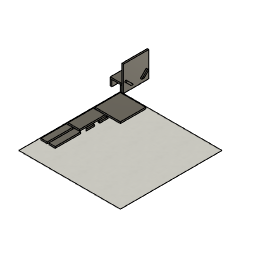
SplineJigV1 (Autodesk Fusion 360 design; units mm, degrees)
Autodesk Fusion 360 part; units mm, degrees
sketch "Sketch2" plane through (0, 0, 0) normal (1, 0, 0) x (0, 1, 0)
  line L0 (0, 0) -> (304.8, 0)
  line L1 (304.8, 0) -> (304.8, 76.2)
  line L2 (304.8, 76.2) -> (0, 76.2)
  line L3 (0, 76.2) -> (0, 0)
  dimension "d1" = 304.8
  dimension "d2" = 76.2
  constraint horizontal L0
  constraint vertical L1
  constraint horizontal L2
  constraint vertical L3
  constraint coincident L0.start L3.end
  measures "d1" distance of L0.start L0.end
  measures "d2" distance of L0.start L2.end
extrude "Extrude1" add sketch "Sketch2" along normal blind 18 makes body 1
sketch "Sketch5" plane through (0, 0, 76.2) normal (0, 0, 1) x (-1, 0, 0)
  line L0 (0, -304.8) -> (0, 0)
  line L1 (0, 0) -> (-18, 0)
  line L2 (-18, 0) -> (-18, -304.8)
  line L3 (-18, -304.8) -> (0, -304.8)
  line L4 (-18, -304.8) -> (121.1875, -304.8)
  line L5 (121.1875, -304.8) -> (121.1875, 0)
  line L6 (121.1875, 0) -> (-18, 0)
  line L7 (-18, 0) -> (-18, -304.8)
  dimension "d11" = 139.1875
  dimension "d12" = 304.8
  constraint horizontal L4
  constraint vertical L5
  constraint horizontal L6
  constraint vertical L7
  constraint coincident L2.end L3.start
  measures "d11" distance of L2.end L4.end
  measures "d12" distance of L2.end L1.end
extrude "Extrude3" add sketch "Sketch5" along normal blind 18 separate body makes body 2
sketch "Sketch6" plane through (0, 0, 76.2) normal (0, 0, -1) x (1, 0, 0)
  line L0 (18, -304.8) -> (18, 0)
  line L1 (18, 0) -> (-121.1875, 0)
  line L2 (-121.1875, 0) -> (-121.1875, -304.8)
  line L3 (-121.1875, -304.8) -> (18, -304.8)
  line L4 (-121.1875, 0) -> (-103.1875, 0)
  line L5 (-103.1875, 0) -> (-103.1875, -304.8)
  line L6 (-103.1875, -304.8) -> (-121.1875, -304.8)
  line L7 (-121.1875, -304.8) -> (-121.1875, 0)
  dimension "d15" = 18
  dimension "d16" = 304.8
  constraint horizontal L4
  constraint vertical L5
  constraint horizontal L6
  constraint vertical L7
  constraint coincident L1.end L2.start
  measures "d15" distance of L1.end L4.end
  measures "d16" distance of L1.end L2.end
extrude "Extrude4" add sketch "Sketch6" along normal blind 76.2 separate body contours L1 L2 L3 L4 L5 L6 L7 makes body 3
sketch "Sketch7" plane through (18, 0, 0) normal (1, 0, 0) x (0, 1, 0)
  line L0 (0, 76.2) -> (0, 0)
  line L1 (0, 0) -> (304.8, 0)
  line L2 (304.8, 0) -> (304.8, 76.2)
  line L3 (304.8, 76.2) -> (0, 76.2)
  line L4 (0, 0) -> (304.8, 0)
  line L5 (304.8, 0) -> (304.8, 304.8)
  line L6 (304.8, 304.8) -> (0, 304.8)
  line L7 (0, 304.8) -> (0, 0)
  dimension "d19" = 304.8
  dimension "d20" = 304.8
  constraint horizontal L4
  constraint vertical L5
  constraint horizontal L6
  constraint vertical L7
  constraint coincident L0.end L1.start
  measures "d19" distance of L0.end L1.end
  measures "d20" distance of L0.end L6.end
extrude "Extrude5" add sketch "Sketch7" along normal blind 18 separate body makes body 4
sketch "Sketch8" plane through (36, 0, 0) normal (1, 0, 0) x (0, 1, 0)
  line L0 (0, 304.8) -> (0, 0)
  line L1 (0, 0) -> (304.8, 0)
  line L2 (304.8, 0) -> (304.8, 304.8)
  line L3 (304.8, 304.8) -> (0, 304.8)
  line L4 (0, 3.175) -> (304.8, 3.175) construction
  line L5 (152.4, 3.175) -> (152.4, 0) construction
  line L6 (152.4, 3.175) -> (304.8, 155.575) construction
  line L7 (152.4, 3.175) -> (368.5341, 3.175) construction
  line L8 (152.4, 3.175) -> (0, 155.575) construction
  line L9 (152.4, 3.175) -> (367.9261, 3.175) construction
  line L10 (203.2, 53.975) -> (275.0421, 125.8171)
  line L11 (275.0421, 125.8171) -> (288.5124, 112.3467)
  line L12 (288.5124, 112.3467) -> (230.1408, 53.975)
  line L13 (101.6, 53.975) -> (29.7579, 125.817)
  line L14 (29.7579, 125.817) -> (16.2876, 112.3467)
  line L15 (16.2876, 112.3467) -> (74.6592, 53.975)
  line L16 (101.6, 53.975) -> (74.6592, 53.975)
  line L17 (203.2, 53.975) -> (230.1408, 53.975)
  dimension "d23" = 3.175
  dimension "d24" = 45
  dimension "d25" = 135
  dimension "d26" = 101.6
  dimension "d29" = 101.6
  dimension "d30" = 19.05
  dimension "d37" = 50.8
  dimension "d38" = 50.8
  dimension "d39" = 19.05
  constraint coincident L0 L4.start
  constraint coincident L2 L4.end
  constraint perpendicular L2 L4
  constraint midpoint L4 L5.start
  constraint midpoint L1 L5.end
  constraint horizontal L7
  constraint coincident L2 L6.end
  constraint horizontal L9
  constraint coincident L0 L8.end
  constraint perpendicular L10 L11
  constraint parallel L10 L12
  constraint coincident L6 L10.end
  constraint parallel L6 L10
  constraint perpendicular L13 L14
  constraint parallel L13 L15
  constraint parallel L8 L13
  constraint coincident L8 L13.start
  constraint horizontal L16
  constraint horizontal L17
  measures "d23" distance of L1 L4
  measures "d24" angle of L6 L7
  measures "d25" angle of L8 L9
  measures "d26" distance of L10.start L10.end
  measures "d29" distance of L13.start L13.end
  measures "d30" distance of L8 L15
  measures "d37" vertical distance of L5.start L10.start
  measures "d38" vertical distance of L5.start L13.start
  measures "d39" distance of L6 L12
extrude "Extrude6" add sketch "Sketch8" along normal blind 18 separate body contours L10 L11 L12 L17 makes body 5
extrude "Extrude7" add sketch "Sketch8" along normal blind 18 separate body contours L13 L14 L15 L16 makes body 6
sketch "Board" plane through (0, 0, 0) normal (0, 0, 1) x (1, 0, 0) in component "Board 1"
  line L0 (0, 0) -> (1219.2, 0)
  line L1 (1219.2, 0) -> (1219.2, -1219.2)
  line L2 (1219.2, -1219.2) -> (0, -1219.2)
  line L3 (0, -1219.2) -> (0, 0)
surface "SurfacePatch1" add patch profiles "Board" section 1 separate body makes body 7 in component "Board 1"
copy_body "CopyPasteBodies1" bodies 4 makes body 8 in component "Body5"
sketch "Body5:1" plane through (0, 0, 0) normal (0, 0, 1) x (1, 0, 0) in component "Board 1"
  line L0 (25.4, -25.4) -> (330.2, -25.4)
  line L1 (330.2, -25.4) -> (330.2, -330.2)
  line L2 (330.2, -330.2) -> (25.4, -330.2)
  line L3 (25.4, -330.2) -> (25.4, -25.4)
  point P0 (177.8, -25.4)
  point P1 (177.8, -330.2)
copy_body "CopyPasteBodies1'" bodies 2 makes body 9 in component "Body3"
sketch "Body3:1" plane through (0, 0, 0) normal (0, 0, 1) x (1, 0, 0) in component "Board 1"
  line L0 (25.4, -349.25) -> (164.592, -349.25)
  line L1 (164.592, -349.25) -> (164.592, -654.05)
  line L2 (164.592, -654.05) -> (25.4, -654.05)
  line L3 (25.4, -654.05) -> (25.4, -349.25)
copy_body "CopyPasteBodies1''" bodies 1 makes body 10 in component "Body1"
sketch "Body1:1" plane through (0, 0, 0) normal (0, 0, 1) x (1, 0, 0) in component "Board 1"
  line L0 (349.25, -25.4) -> (425.45, -25.4)
  line L1 (425.45, -25.4) -> (425.45, -330.2)
  line L2 (425.45, -330.2) -> (349.25, -330.2)
  line L3 (349.25, -330.2) -> (349.25, -25.4)
copy_body "CopyPasteBodies1'''" bodies 3 makes body 11 in component "Body4"
sketch "Body4:1" plane through (0, 0, 0) normal (0, 0, 1) x (1, 0, 0) in component "Board 1"
  line L0 (25.4, -673.1) -> (101.6, -673.1)
  line L1 (101.6, -673.1) -> (101.6, -977.9)
  line L2 (101.6, -977.9) -> (25.4, -977.9)
  line L3 (25.4, -977.9) -> (25.4, -673.1)
copy_body "CopyPasteBodies1''''" bodies 5 makes body 12 in component "Body6"
sketch "Body6:1" plane through (0, 0, 0) normal (0, 0, 1) x (1, 0, 0) in component "Board 1"
  line L0 (183.642, -349.25) -> (202.692, -349.25)
  line L1 (202.692, -349.25) -> (202.692, -450.85)
  line L2 (202.692, -450.85) -> (183.642, -450.85)
  line L3 (183.642, -450.85) -> (183.642, -349.25)
copy_body "CopyPasteBodies1'''''" bodies 6 makes body 13 in component "Body7"
sketch "Body7:1" plane through (0, 0, 0) normal (0, 0, 1) x (1, 0, 0) in component "Board 1"
  line L0 (349.25, -349.25) -> (368.3, -349.25)
  line L1 (368.3, -349.25) -> (368.3, -450.85)
  line L2 (368.3, -450.85) -> (349.25, -450.85)
  line L3 (349.25, -450.85) -> (349.25, -349.25)
move_body "Move1" bodies 10 to x (1, 0, 0) y (0, 1, 0) z (0, 0, 1) at (0, -647.6962, -228.5941) in component "Body1"
move_body "Move1'" bodies 12 to x (0, 0.707107, -0.707107) y (-0.707107, 0.5, 0.5) z (0.707107, 0.5, 0.5) at (169.568, 49.1507, -49.1507) in component "Body6"
move_body "Move1''" bodies 13 to x (0, -0.707107, -0.707107) y (0.707107, 0.5, -0.5) z (0.707107, -0.5, 0.5) at (-190.7381, 218.1966, -11.698) in component "Body7"
move_body "Move2" bodies 12 to x (1, 0, 0) y (0, 1, 0) z (0, 0, 1) at (-9.525, 0, 0) in component "Body6"
move_body "Move2'" bodies 13 to x (1, 0, 0) y (0, 1, 0) z (0, 0, 1) at (-30.353, 0, 0) in component "Body7"
component "map" placed x (1, 0, 0) y (0, 1, 0) z (0, 0, 1) at (0, 0, 0)
component "linked" placed x (1, 0, 0) y (0, 1, 0) z (0, 0, 1) at (0, 0, 0) in component "map"
component "Board 1" placed x (1, 0, 0) y (0, 1, 0) z (0, 0, 1) at (0, 0, 0) in component "map"
component "Body5" placed x (0, 0, -1) y (0, 1, 0) z (1, 0, 0) at (25.4, -330.2, 36) in component "Board 1"
component "Body3" placed x (1, 0, 0) y (0, -1, 0) z (0, 0, -1) at (146.5898, -349.25, 94.2) in component "Board 1"
component "Body1" placed x (0, 0, -1) y (0, 1, 0) z (1, 0, 0) at (349.25, -330.2, 18) in component "Board 1"
component "Body4" placed x (0, 0, 1) y (0, -1, 0) z (1, 0, 0) at (25.4, -673.1, 121.1875) in component "Board 1"
component "Body6" placed x (1, 0, 0) y (0, -0.707107, 0.707107) z (0, -0.707107, -0.707107) at (148.167, -167.3998, -105.518) in component "Board 1"
component "Body7" placed x (1, 0, 0) y (0, -0.707107, -0.707107) z (0, 0.707107, -0.707107) at (313.775, -417.174, 110.0081) in component "Board 1"
equation "d1 = length"
equation "d2 = fenceHeight"
equation "d3 = thickness"
equation "d11 = fenceWidth + thickness * 2"
equation "d12 = length"
equation "d13 = thickness"
equation "d15 = thickness"
equation "d16 = length"
equation "d17 = fenceHeight"
equation "d19 = length"
equation "d20 = height"
equation "d21 = thickness"
equation "d30 = ( 3 / 4 ) * 1 in"
equation "d32 = thickness"
equation "d34 = thickness"
equation "d37 = angleHeight"
equation "d38 = angleHeight"
equation "MapMapType = 0"
equation "MapLaserKerf = 0"
equation "MapLineThickness = 1"
equation "MapSVGScale = 0"
equation "MapLineColors = 1" comment "5,1,3,8"
equation "MapBoardDXF = 0"
equation "MapBoardSVG = 0"
equation "MapCutouts = 1"
equation "MapInsets = 1"
equation "MapSvgLabels = 1"
equation "MapSheets = 1"
equation "MapNesting = 0"
equation "MapArrangeType = 2"
equation "MapKerf = 1.905"
equation "MapEdgeTrim = 2.54"
equation "MapIgnoreThickness = 0"
equation "MapCutlist = 0"
equation "MapLabels = 0"
equation "MapFont = 1" comment "Arial"
equation "MapBoardLabelSize = 0"
equation "MapCompLabelSize = 0"
equation "MapOrientation = 0"
equation "MapUseAppearance = 0"
equation "MapCanRotate = 1"
equation "MapGlass = 0"
equation "MapLogLevel = 20"
equation "MapBoard0 = 1" comment "Steel:121.92:121.92:1.800"
equation "angle = 0.0 deg"
equation "offset = 0.00 in"
equation "thickness = 18 mm"
equation "fenceHeight = 3 in"
equation "length = 12 in"
equation "fenceWidth = 4 in + ( 1 / 16 ) * 1 in"
equation "height = 12 in"
equation "angleHeight = 2 in"
named bodies: "Board 1 [1.800]", "Body5", "Body3", "Body1", "Body4", "Body6", "Body7"
